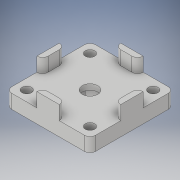
# Autodesk Inventor part: feet_screw_adapter
Saved by Autodesk Inventor 2019 (Build 230136000, 136)
## iProperties
Created: 2018-05-26
Part Number: feet_screw_adapter
Material: Generisch
Document SubType Name: Modeling
Designer: marc
Density: 1 g/cm^3
Appearance: Vorgabe
Author: marc
## iProperties of the stored document feet_screw_adapter_3D-Druck.ipt
Created: 2018-05-26
Part Number: feet_screw_adapter_3D-Druck
Material: Generisch
Document SubType Name: Modeling
Designer: marc
Density: 1 g/cm^3
Appearance: Vorgabe
Author: marc
Autodesk Inventor part; units mm, degrees
ref_plane "YZ Plane" through (0, 0, 0) normal (1, 0, 0) x (0, 1, 0)
ref_plane "XZ Plane" through (0, 0, 0) normal (0, 1, 0) x (-1, 0, 0)
ref_plane "XY Plane" through (0, 0, 0) normal (0, 0, 1) x (1, 0, 0)
sketch "Skizze1" plane through (0, 0, 0) normal (0, 1, 0) x (-1, 0, 0)
  line L0 (0, 0) -> (30, 0)
  line L1 (30, 0) -> (30, 30)
  line L2 (30, 30) -> (0, 30)
  line L3 (0, 30) -> (0, 0)
  dimension "d0" = 30
  dimension "d1" = 30
  constraints: 8 end point, 2 parallel, 1 horizontal, 1 perpendicular
  measures "d0" distance of L2.end L1.end
  measures "d1" distance of L1.end L0.end
extrude "Extrusion1" add sketch "Skizze1" along normal blind 5
sketch "Skizze2" plane through (0, 5, 0) normal (0, 1, 0) x (1, 0, 0)
  line L0 (-30, -19) -> (-28, -19)
  line L1 (-28, -19) -> (-28, -11)
  line L2 (-28, -11) -> (-30, -11)
  line L3 (-30, -11) -> (-30, -19)
  line L4 (-19, -2) -> (-11, -2)
  line L5 (-11, -2) -> (-11, 0)
  line L6 (-11, 0) -> (-19, 0)
  line L7 (-19, 0) -> (-19, -2)
  line L8 (-2, -19) -> (0, -19)
  line L9 (0, -19) -> (0, -11)
  line L10 (0, -11) -> (-2, -11)
  line L11 (-2, -11) -> (-2, -19)
  line L12 (-19, -30) -> (-11, -30)
  line L13 (-11, -30) -> (-11, -28)
  line L14 (-11, -28) -> (-19, -28)
  line L15 (-19, -28) -> (-19, -30)
  line L16 (-30, 0) -> (-30, -30) projected
  line L17 (0, 0) -> (-30, 0) projected
  line L18 (0, -30) -> (0, 0) projected
  line L19 (-30, -30) -> (0, -30) projected
  dimension "d4" = 0
  dimension "d5" = 0
  dimension "d6" = 0
  dimension "d7" = 0
  dimension "d8" = 2
  dimension "d9" = 8
  dimension "d10" = 11
  dimension "d11" = 11
  dimension "d12" = 11
  constraints: 32 end point, 8 parallel, 5 equal length, 4 horizontal, 4 perpendicular, 2 point on line
  measures "d4" distance between parallel lines of L16 L3
  measures "d5" distance between parallel lines of L17 L6
  measures "d6" distance between parallel lines of L18 L9
  measures "d7" distance between parallel lines of L19 L12
  measures "d8" distance of L12.end L13.end
  measures "d9" distance of L10.end L8.start
  measures "d10" distance between parallel lines of L17 L2
  measures "d11" distance between parallel lines of L16 L7
  measures "d12" distance between parallel lines of L17 L10
extrude "Extrusion2" add sketch "Skizze2" along normal blind 5 contours L3 L2 L1 L0 | L15 L14 L13 L12 | L6 L5 L4 L7 | L8 L11 L10 L9
sketch "Skizze3" plane through (0, 5, 0) normal (0, 1, 0) x (1, 0, 0)
  line L0 (0, -30) -> (0, -19) projected
  line L1 (-11, -30) -> (0, -30) projected
  line L2 (0, 0) -> (-11, 0) projected
  line L3 (0, -11) -> (0, 0) projected
  line L4 (-30, -19) -> (-30, -30) projected
  line L5 (-30, -30) -> (-19, -30) projected
  line L6 (-30, 0) -> (-30, -11) projected
  line L7 (-19, 0) -> (-30, 0) projected
  point P0 (-26.3, -26.3)
  point P1 (-26.3, -3.7)
  point P2 (-3.7, -3.7)
  point P3 (-3.7, -26.3)
  dimension "d15" = 3.7
  dimension "d16" = 3.7
  dimension "d17" = 3.7
  dimension "d18" = 3.7
  dimension "d19" = 3.7
  dimension "d20" = 3.7
  dimension "d21" = 3.7
  dimension "d22" = 3.7
  measures "d15" distance from line of L0 point (-3.7, -26.3)
  measures "d16" distance from line of L1 point (-3.7, -26.3)
  measures "d17" distance from line of L2 point (-3.7, -3.7)
  measures "d18" distance from line of L3 point (-3.7, -3.7)
  measures "d19" distance from line of L4 point (-26.3, -26.3)
  measures "d20" distance from line of L5 point (-26.3, -26.3)
  measures "d21" distance from line of L6 point (-26.3, -3.7)
  measures "d22" distance from line of L7 point (-26.3, -3.7)
hole "Bohrung1" at (-26.3, 5, 26.3) at (-26.3, 5, 3.7) at (-3.7, 5, 3.7) at (-3.7, 5, 26.3) direction (0, -1, 0) diameter 3.4 end through all
sketch "Skizze4" plane through (0, 5, 0) normal (0, 1, 0) x (1, 0, 0)
  line L0 (-19, 0) -> (-30, 0) projected
  line L1 (0, -11) -> (0, 0) projected
  point P0 (-15, -15)
  dimension "d30" = 15
  dimension "d31" = 15
  measures "d30" distance from line of L0 point (-15, -15)
  measures "d31" distance from line of L1 point (-15, -15)
hole "Bohrung2" at (-15, 5, 15) direction (0, -1, 0) diameter 5.5 end through all clearance for "Flachkopfsenkschraube DIN EN ISO 2009" size "M5" standard "DIN"
sketch "Skizze6" plane through (0, 0, 0) normal (0, -1, 0) x (1, 0, 0)
  line L0 (0, 0) -> (-30, 0) projected
  line L1 (0, 30) -> (0, 0) projected
  line L2 (-11.05, 17.2805) -> (-11.05, 12.7195)
  line L3 (-11.05, 12.7195) -> (-15, 10.4389)
  line L4 (-15, 10.4389) -> (-18.95, 12.7195)
  line L5 (-18.95, 12.7195) -> (-18.95, 17.2805)
  line L6 (-18.95, 17.2805) -> (-15, 19.5611)
  line L7 (-15, 19.5611) -> (-11.05, 17.2805)
  point P0 (-15, 15)
  point P1 (-15, 15)
  dimension "d41" = 15
  dimension "d42" = 15
  dimension "d43" = 7.9
  constraints: 12 end point, 1 coincident, 1 parallel, 13 other
  measures "d41" distance from line of L0 point (-15, 15)
  measures "d42" distance from line of L1 point (-15, 15)
  measures "d43" distance between parallel lines of L5 L2
extrude "Extrusion3" cut sketch "Skizze6" against normal blind 3
fillet "Rundung1" radius 2 12 edges at (-30, 2.5, 0) (0, 2.5, 0) (-30, 2.5, 30) (0, 2.5, 30) (-11, 7.5, 28) (-19, 7.5, 28) (-28, 7.5, 19) (-28, 7.5, 11) (-2, 7.5, 19) (-2, 7.5, 11) (-19, 7.5, 2) (-11, 7.5, 2)
equation "\"d17\" = d16"
equation "\"d18\" = d15"
equation "\"d19\" = d15"
equation "\"d20\" = d16"
equation "\"d21\" = d15"
equation "\"d22\" = d16"
